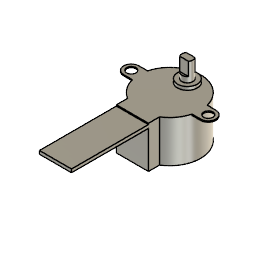
Oct 24 Cup Drawing Machine (Autodesk Fusion 360 archive; units mm, degrees)
design "Step Motor ref"
Autodesk Fusion 360 part; units mm, degrees
sketch "Sketch1" plane through (0, 0, 0) normal (0, 0, 1) x (1, 0, 0)
  line L0 (0, 0) -> (-17.5, 0)
  circle A0 centre (-17.5, 0) radius 2.1
  line L1 (0, 14) -> (0, 8)
  circle A1 centre (0, 8) radius 4.5
  circle A2 centre (0, 8) radius 2.5
  circle A3 centre (0, 8) radius 1.5 construction
  line L2 (-2, 9.5) -> (2, 9.5)
  line L3 (-2, 6.5) -> (2, 6.5)
  line L4 (-13.5554, 3.5) -> (-17.5, 3.5)
  arc A4 (-17.5, 3.5) -> (-17.5, -3.5) centre (-17.5, 0) ccw
  line L5 (-17.5, -3.5) -> (-13.5554, -3.5)
  line L6 (13.5554, 3.5) -> (17.5, 3.5)
  arc A5 (17.5, -3.5) -> (17.5, 3.5) centre (17.5, 0) ccw
  line L7 (17.5, -3.5) -> (13.5554, -3.5)
  circle A6 centre (17.5, 0) radius 2.1
  line L8 (-7.3, 0) -> (7.3, 0)
  line L9 (7.3, 0) -> (7.3, -17)
  line L10 (7.3, -17) -> (-7.3, -17)
  line L11 (-7.3, -17) -> (-7.3, 0)
  circle A7 centre (0, 0) radius 14
  line L12 (-7.3, -17) -> (7.3, -17)
  line L13 (7.3, -17) -> (7.3, -52)
  line L14 (7.3, -52) -> (-7.3, -52)
  line L15 (-7.3, -52) -> (-7.3, -17)
  dimension "d1" = 17.5
  dimension "d2" = 28
  dimension "d3" = 4.2
  dimension "d5" = 9
  dimension "d6" = -2
  dimension "d7" = -3
  dimension "d8" = 7
  dimension "d9" = 17
  dimension "d10" = 14.6
  dimension "d19" = 8
  dimension "d22" = 35
  constraint coincident L0.start A7.centre
  constraint horizontal L0
  constraint coincident L0.end A0.centre
  constraint perpendicular L0 L1
  constraint coincident L1.end A1.centre
  constraint coincident A2 L2.start
  constraint coincident A2 L2.end
  constraint perpendicular L1 L2
  constraint coincident A2 L3.start
  constraint coincident A2 L3.end
  constraint perpendicular L1 L3
  constraint tangent A3 L2
  constraint tangent A3 L3
  constraint horizontal L4
  constraint tangent L4 A4
  constraint coincident L5.end A7
  constraint parallel L4 L5
  constraint symmetric L0 L4 L5
  constraint tangent A4 L5
  constraint concentric A0 A4
  constraint symmetric A0 L1 A6
  constraint symmetric L1 L4.start L6.start
  constraint symmetric L1 L4.end L6.end
  constraint symmetric L1 A4.end A5.start
  constraint symmetric L1 A4 A5
  constraint symmetric L1 L5.end L7.end
  constraint horizontal L8
  constraint vertical L9
  constraint horizontal L10
  constraint vertical L11
  constraint coincident L0 L8.start
  constraint coincident L4.start A7
  constraint coincident L6.start A7
  constraint coincident L7.end A7
  constraint coincident L1.start A7
  constraint horizontal L12
  constraint vertical L13
  constraint horizontal L14
  constraint vertical L15
  constraint collinear L9 L13
  measures "d1" distance of L0.start L0.end
  measures "d2" diameter of A7
  measures "d3" diameter of A0
  measures "d5" diameter of A1
  measures "d8" distance of L4 L5
  measures "d9" distance of L8 L10
  measures "d10" distance of L9 L11
  measures "d19" distance of L0.start L1.end
  measures "d22" distance of L10 L14
extrude "Extrude1" add sketch "Sketch1" against normal blind 19 contours L0 L8 L9 L11 A7 | L0 L8 L9 A7 | L0 L11 A7 | L9 L10 L11 A7 L12 | L1 A2 L2 | L1 A2 L2 | A2 L2 L3 | A2 L3 | A1
extrude "Extrude2" add sketch "Sketch1" along normal blind 10 contours A2 L2 L3
extrude "Extrude3" add sketch "Sketch1" along normal blind 4 contours L1 A2 L2 | L1 A2 L2 | A2 L3
extrude "Extrude4" add sketch "Sketch1" along normal blind 1.5 contours A1
extrude "Extrude5" add sketch "Sketch1" against normal blind 0.5 contours L4 A4 L5 A7 | L6 A5 L7 A7
extrude "Extrude6" add sketch "Sketch1" against normal blind 1.5 from surface at -0.5 contours L10 L12 L13 L14 L15
equation "d1 = ( 35 / 2 ) * 1 mm"
